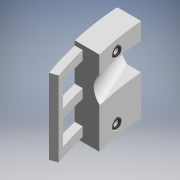
# Autodesk Inventor part: 4978445 CMMT-AS-3A---(clamp)
Saved by Autodesk Inventor 2017.3 (Build 213256000, 256)
## iProperties
Part Number: 4978445 CMMT-AS-3A---(clamp)
Material: Generic
Catalog Web Link: www.cadenas.de
Description: CMMT-clamp-Shield clamp
Vendor: FESTO
Document SubType Name: Modeling
Designer: partserver
Manufacturer: FESTO
Mass: 15.0748 g
Surface Area: 64.8567 cm^2
Volume: 15.0748 cm^3
Density: 1 g/cm^3
Appearance: PSOLRGB-255-255-255
Category: PARTsolutions
Company: FESTO
Title: 4978445 CMMT-AS-3A---(clamp)
Author: Cadenas PARTsolutions
Comments: Shield clamp
PSOL_IDENT_0: {$CADENAS_DATA\23d-libs\festo\parts\c\cmmt\parts\cmmt_clamp.prj},200 {VTYP=3D},{NB=4978445 CMMT-AS-3
PSOL_IDENT_1: A---(clamp)},{LINA=4978445 CMMT-AS-3A---(clamp)},{NN=CMMT-clamp},{DATE=07.10.2020 06:56:02},{GEOMDAT
PSOL_IDENT_2: E=07.10.2020 06:45:00},{VERSION=},{LINEID=10},{WBVAR=},{WBNUMERIC=}  {NB=4978445 CMMT-AS-3A---(clamp
PSOL_IDENT_3: )},{LINA=4978445 CMMT-AS-3A---(clamp)},{KT=DUMMY},{TNR=4978445},{TYP=CMMT-AS-3A},{B1=45.800},{B2=13.
PSOL_IDENT_4: 000},{B3=34.000},{H1=47.100},{H2=27.200},{R1=175.500},{B4=13.050},{H3=15.200}
NB: 4978445 CMMT-AS-3A---(clamp)
NN: CMMT-clamp
NT: Shield clamp
NBSYN: $TNR. $TYP.---(clamp)
LINA: 4978445 CMMT-AS-3A---(clamp)
CATALOG: Festo
TNR: 4978445
TYP: CMMT-AS-3A
B1: 45.8
B2: 13
B3: 34
H1: 47.1
H2: 27.2
R1: 175.5
B4: 13.05
H3: 15.2
SUPPLIER: FESTO
ARTICLENO: 4978445 CMMT-AS-3A---(clamp)
BOMINFO: 4978445 CMMT-AS-3A---(clamp)
CREATOR: CADENAS GmbH
Autodesk Inventor part; units mm, degrees
sketch "Sketch_1" plane through (0, 0, 0) normal (0, 0, 1) x (1, 0, 0)
  arc A0 (-4.4213, -26.8889) -> (-4.1788, -27.2) centre (-4.1788, -26.95) ccw
  line L0 (-4.1788, -27.2) -> (4.658, -27.2)
  arc A1 (-0.814, -45.4529) -> (4.658, -27.2) centre (-162.0052, 12.8168) ccw
  arc A2 (-0.814, -45.4529) -> (-0.6644, -45.7728) centre (-0.5789, -45.5379) ccw
  line L1 (-0.6644, -45.7728) -> (2.982, -47.1)
  arc A3 (2.982, -47.1) -> (13.0099, -0.538) centre (-161.9834, 12.7889) ccw
  arc A4 (13.0099, -0.538) -> (12.5113, 0) centre (12.5113, -0.5) ccw
  line L2 (12.5113, 0) -> (0.2308, 0)
  arc A5 (0.2308, 0) -> (-0.0184, -0.2299) centre (0.2308, -0.25) ccw
  arc A6 (-4.4213, -26.8889) -> (-0.0184, -0.2299) centre (-161.9929, 12.828) ccw
  constraints: 14 point on circle, 7 centre point, 6 end point
extrude "Extrusion1" add sketch "Sketch_1" along normal mid plane 45.8
sketch "Sketch_2" plane through (0, 0, 0) normal (1, 0, 0) x (0, 1, 0)
  line L0 (-27.4, 15.5) -> (-42, 15.5)
  arc A0 (-42, 15.5) -> (-42.2, 15.3) centre (-42, 15.3) ccw
  line L1 (-42.2, 15.3) -> (-42.2, 2.7)
  arc A1 (-42.2, 2.7) -> (-42, 2.5) centre (-42, 2.7) ccw
  line L2 (-42, 2.5) -> (-27.4, 2.5)
  arc A2 (-27.4, 2.5) -> (-27.2, 2.7) centre (-27.4, 2.7) ccw
  line L3 (-27.2, 2.7) -> (-27.2, 15.3)
  arc A3 (-27.2, 15.3) -> (-27.4, 15.5) centre (-27.4, 15.3) ccw
  constraints: 8 end point, 8 point on circle, 4 centre point
extrude "Extrusion2" cut sketch "Sketch_2" along normal blind 15
sketch "Sketch_3" plane through (0, 0, 0) normal (1, 0, 0) x (0, 1, 0)
  arc A0 (-42, -2.5) -> (-42.2, -2.7) centre (-42, -2.7) ccw
  line L0 (-42.2, -2.7) -> (-42.2, -15.3)
  arc A1 (-42.2, -15.3) -> (-42, -15.5) centre (-42, -15.3) ccw
  line L1 (-42, -15.5) -> (-27.4, -15.5)
  arc A2 (-27.4, -15.5) -> (-27.2, -15.3) centre (-27.4, -15.3) ccw
  line L2 (-27.2, -15.3) -> (-27.2, -2.7)
  arc A3 (-27.2, -2.7) -> (-27.4, -2.5) centre (-27.4, -2.7) ccw
  line L3 (-27.4, -2.5) -> (-42, -2.5)
  constraints: 8 end point, 8 point on circle, 4 centre point
extrude "Extrusion3" cut sketch "Sketch_3" along normal blind 15
sketch "Sketch_4" plane through (13.01, 0, 0) normal (1, 0, 0) x (0, 0, -1)
  line L0 (-22.9, -47.1) -> (-20.5, -47.1)
  line L1 (-20.5, -47.1) -> (-20.5, -27.2)
  line L2 (-20.5, -27.2) -> (-22.9, -27.2)
  line L3 (-22.9, -27.2) -> (-22.9, -47.1)
  constraints: 8 end point
extrude "Extrusion4" cut sketch "Sketch_4" along normal mid plane 40
sketch "Sketch_5" plane through (13.01, 0, 0) normal (1, 0, 0) x (0, 0, -1)
  line L0 (20.5, -47.1) -> (22.9, -47.1)
  line L1 (22.9, -47.1) -> (22.9, -27.2)
  line L2 (22.9, -27.2) -> (20.5, -27.2)
  line L3 (20.5, -27.2) -> (20.5, -47.1)
  constraints: 8 end point
extrude "Extrusion5" cut sketch "Sketch_5" along normal mid plane 30
sketch "Sketch_6" plane through (0, -15.2, 0) normal (0, 1, 0) x (1, 0, 0)
  line L0 (-3, -17) -> (13.65, -17)
  line L1 (13.65, -17) -> (13.65, -21)
  line L2 (13.65, -21) -> (6.9, -21)
  arc A0 (6.65, -20.75) -> (6.9, -21) centre (6.9, -20.75) ccw
  line L3 (6.65, -20.75) -> (6.65, -19.25)
  line L4 (6.65, -19.25) -> (-1.2, -19.5241)
  line L5 (-1.2, -19.5241) -> (-1.2, -20)
  line L6 (-1.2, -20) -> (-3, -20)
  line L7 (-3, -20) -> (-3, -17)
  line L8 (-3, -17) -> (13.65, -17)
  constraints: 18 end point, 2 point on circle, 1 centre point
revolve "Revolution1" cut sketch "Sketch_6" angle 360 about axis through (-3, -15.2, 17) along (-1, 0, 0)
sketch "Sketch_7" plane through (0, -15.2, 0) normal (0, 1, 0) x (1, 0, 0)
  line L0 (-3, 17) -> (13.65, 17)
  line L1 (13.65, 17) -> (13.65, 13)
  line L2 (13.65, 13) -> (6.9, 13)
  arc A0 (6.65, 13.25) -> (6.9, 13) centre (6.9, 13.25) ccw
  line L3 (6.65, 13.25) -> (6.65, 14.75)
  line L4 (6.65, 14.75) -> (-1.2, 14.4759)
  line L5 (-1.2, 14.4759) -> (-1.2, 14)
  line L6 (-1.2, 14) -> (-3, 14)
  line L7 (-3, 14) -> (-3, 17)
  line L8 (-3, 17) -> (13.65, 17)
  constraints: 18 end point, 2 point on circle, 1 centre point
revolve "Revolution2" cut sketch "Sketch_7" angle 360 about axis through (-3, -15.2, -17) along (-1, 0, 0)
sketch "Sketch_8" plane through (0, -15.2, 0) normal (0, 1, 0) x (1, 0, 0)
  line L0 (-2.1, -17) -> (-0.9, -17)
  circle A0 centre (-1.5, -19.1) radius 0.6
  constraints: 2 end point, 1 centre point
revolve "Revolution3" add sketch "Sketch_8" angle 360 about axis through (-2.1, -15.2, 17) along (-1, 0, 0)
sketch "Sketch_13" plane through (0, -15.2, 0) normal (0, 1, 0) x (1, 0, 0)
  line L0 (-2.1, 17) -> (-0.9, 17)
  circle A0 centre (-1.5, 14.9) radius 0.6
  constraints: 2 end point, 1 centre point
revolve "Revolution4" add sketch "Sketch_13" angle 360 about axis through (-2.1, -15.2, -17) along (-1, 0, 0)
sketch "Sketch_11" plane through (-2.1131, -31.7315, 0) normal (0.4226, 0.9063, 0) x (0.9063, -0.4226, 0)
  line L0 (-14.5, -1.3) -> (-4.5, -1.3)
  line L1 (-4.5, -1.3) -> (-3.2407, 0.2007)
  arc A0 (-3.2407, 0.2007) -> (-3.2407, 12.1993) centre (-11.428, 6.2) ccw
  line L2 (-3.2407, 12.1993) -> (-4.5, 13.7)
  line L3 (-4.5, 13.7) -> (-14.5, 13.7)
  line L4 (-14.5, 13.7) -> (-14.5, -1.3)
  constraints: 10 end point, 2 point on circle, 1 centre point
extrude "Extrusion6" cut sketch "Sketch_11" along normal blind 35
ref_plane "ANBAU_XY" through (0, 0, 0) normal (1, 0, 0) x (0, 0, -1)
ref_plane "ANBAU_YZ" through (0, 0, 0) normal (0, 0, -1) x (0, 1, 0)
ref_plane "ANBAU_ZX" through (0, 0, 0) normal (0, 1, 0) x (1, 0, 0)
ref_plane "SCREW_1_XY" through (6.65, -15.2, 17) normal (1, 0, 0) x (0, 0, -1)
ref_plane "SCREW_1_YZ" through (6.65, -15.2, 17) normal (0, 0, -1) x (0, 1, 0)
ref_plane "SCREW_1_ZX" through (6.65, -15.2, 17) normal (0, 1, 0) x (1, 0, 0)
ref_plane "SCREW_2_XY" through (6.65, -15.2, -17) normal (1, 0, 0) x (0, 0, -1)
ref_plane "SCREW_2_YZ" through (6.65, -15.2, -17) normal (0, 0, -1) x (0, 1, 0)
ref_plane "SCREW_2_ZX" through (6.65, -15.2, -17) normal (0, 1, 0) x (1, 0, 0)
body "Solid1"
